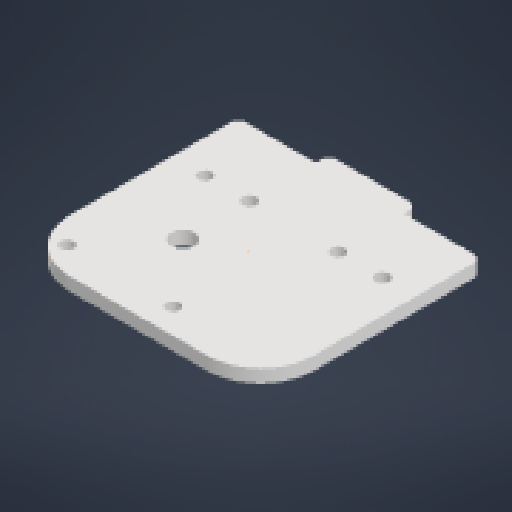
# Autodesk Inventor part: PlacaBaseGarraPotenciaSTD
Saved by Autodesk Inventor 2026.3 (Build 303398000, 398)
## iProperties
Created: 2026-04-16
Part Number: PlacaBaseGarraPotenciaSTD
Material: Genérico
Document SubType Name: Modeling
Designer: Jose Carlos
Density: 1 g/cm^3
Appearance: Valor por defecto
Author: Jose Carlos
Autodesk Inventor part; units mm, degrees
ref_plane "YZ Plane" through (0, 0, 0) normal (1, 0, 0) x (0, 1, 0)
ref_plane "XZ Plane" through (0, 0, 0) normal (0, 1, 0) x (-1, 0, 0)
ref_plane "XY Plane" through (0, 0, 0) normal (0, 0, 1) x (1, 0, 0)
sketch "Boceto1" plane through (0, 0, 0) normal (0, 1, 0) x (-1, 0, 0)
  line L0 (27.5, 25) -> (-27.5, 25)
  line L1 (-27.5, 25) -> (-27.5, -25)
  line L2 (-27.5, -25) -> (27.5, -25)
  line L3 (27.5, -25) -> (27.5, 25)
  line L4 (27.5, 25) -> (-27.5, -25) construction
  line L5 (-27.5, 25) -> (27.5, -25) construction
  point P0 (0, 0)
  dimension "d0" = 55
  dimension "d1" = 50
  constraints: 12 end point, 2 midpoint, 2 parallel, 1 horizontal, 1 perpendicular
  measures "d0" distance of L1.end L2.end
  measures "d1" distance of L2.end L0.start
extrude "Extrusión1" add sketch "Boceto1" along normal blind 3
sketch "Boceto2" plane through (0, 3, 0) normal (0, 1, 0) x (1, 0, 0)
  line L0 (10, 22) -> (-10, 22)
  line L1 (-10, 22) -> (-10, 28)
  line L2 (-10, 28) -> (10, 28)
  line L3 (10, 28) -> (10, 22)
  line L4 (27.5, 25) -> (-27.5, 25) construction
  line L5 (10, 22) -> (-10, 28) construction
  line L6 (-10, 22) -> (10, 28) construction
  point P0 (0, 0)
  point P1 (0, 25)
  dimension "d4" = 6
  dimension "d5" = 20
  constraints: 12 end point, 3 midpoint, 2 parallel, 1 horizontal, 1 perpendicular
  measures "d4" distance of L0.end L1.end
  measures "d5" distance of L1.end L2.end
extrude "Extrusión2" add sketch "Boceto2" against normal blind 3
fillet "Empalme1" radius 2 4 edges at (-27.5, 1.5, -25) (-10, 1.5, -28) (10, 1.5, -28) (27.5, 1.5, -25)
sketch "Boceto3" plane through (0, 3, 0) normal (0, 1, 0) x (1, 0, 0)
  circle A0 centre (-20, 10) radius 1.6 construction
  circle A1 centre (-10, -5) radius 1.5 construction
  circle A2 centre (-10, 10) radius 1.6 construction
  line L0 (0, 38.6) -> (0, -35.6) construction
  circle A3 centre (20, 10) radius 1.6 construction
  circle A4 centre (10, 10) radius 1.6 construction
  circle A5 centre (-22, -19.2272) radius 1.7 construction
  circle A6 centre (2, -19.2272) radius 1.7 construction
  point P0 (0, 0)
  constraints: 5 coincident, 4 symmetric about line, 2 centre point, 2 other
hole "Agujero1" at (-20, 3, -10) at (-10, 3, -10) at (10, 3, -10) at (20, 3, -10) at (2, 3, 19.2272) at (-22, 3, 19.2272) direction (0, -1, 0) diameter 3 end through all
sketch "Boceto4" plane through (0, 3, 0) normal (0, 1, 0) x (1, 0, 0)
  circle A0 centre (-10, -5) radius 1.5 construction
  point P0 (0, 0)
  constraints: 1 coincident
hole "Agujero2" at (-10, 3, 5) direction (0, -1, 0) diameter 5.2 end through all
fillet "Empalme2" radius 12 2 edges at (27.5, 1.5, 25) (-27.5, 1.5, 25)
